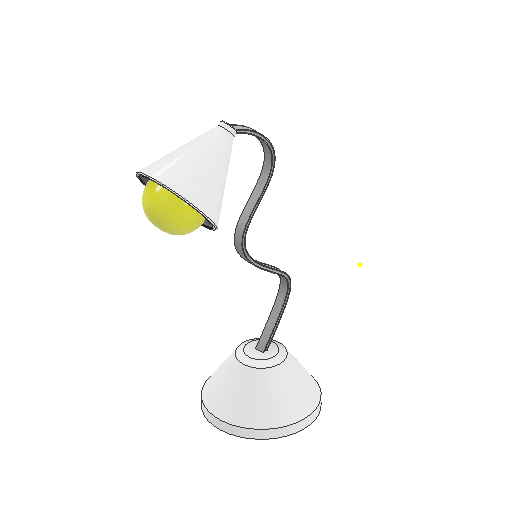
# Autodesk Inventor part: Lamp
Saved by Autodesk Inventor 2026.2 (Build 302298000, 298)
## iProperties
Created: 2026-01-20
Part Number: Lamp
Material: Generic
Document SubType Name: Modeling
Designer: andyeske
Density: 1 g/cm^3
Appearance: Default
Author: andyeske
Autodesk Inventor part; units mm, degrees
ref_plane "YZ Plane" through (0, 0, 0) normal (1, 0, 0) x (0, 1, 0)
ref_plane "XZ Plane" through (0, 0, 0) normal (0, 1, 0) x (-1, 0, 0)
sketch "Sketch1" plane through (0, 0, 0) normal (0, 0, 1) x (1, 0, 0)
  line L0 (0, 0) -> (14.1629, 0)
  line L1 (14.1629, 0) -> (14.1629, 2.8634)
  line L2 (14.1629, 2.8634) -> (5.4597, 15.9183)
  line L3 (5.4597, 15.9183) -> (0, 15.9183)
  line L4 (0, 15.9183) -> (0, 0)
  constraints: 10 end point, 2 perpendicular, 1 horizontal, 1 parallel
revolve "Revolution1" add sketch "Sketch1" angle 360 about axis through (0, 15.9183, 0) along (0, -1, 0)
sketch "Sketch2" plane through (0, 0, 0) normal (1, 0, 0) x (0, 1, 0)
  line L0 (15.9183, 5.4597) -> (15.9183, -5.4597) projected
  spline S0 degree 4 poles (15.9183, 0) (34.1677, -12.4464) (32.4638, -9.3286) (51.0132, 21.4952) (65.6277, -11.3456) (81.7247, 0.6772) (85.1054, 10.9604) (85.0776, 11.7877) knots 0 0 0 0 0 0.334349 0.547583 0.739077 1 1 1 1 1
  line L1 (-0.0819, 10.9124) -> (31.9186, -10.9124) construction
  arc A0 (3.2241, 8.8777) -> (28.8174, -8.5773) centre (387.7406, 545.1818) ccw construction
  line L2 (85.1268, 10.3231) -> (85.0285, 13.2523) construction
  arc A1 (84.8109, 11.3786) -> (84.7841, 12.178) centre (84.6524, 11.7734) ccw construction
  point P0 (0, 0)
  point P1 (37.5795, -3.3142)
  point P2 (52.1302, 7.0993)
  point P3 (67.4583, -2.4293)
  point P4 (81.2439, 4.0296)
  constraints: 5 midpoint, 4 end point, 2 centre point, 2 point on circle, 10 other
sketch "Sketch3" plane through (0, 15.9183, 0) normal (0, 1, 0) x (1, 0, 0)
  line L0 (1.27, -0.635) -> (-1.27, -0.635)
  line L1 (-1.27, -0.635) -> (-1.27, 0.635)
  line L2 (-1.27, 0.635) -> (1.27, 0.635)
  line L3 (1.27, 0.635) -> (1.27, -0.635)
  line L4 (1.27, -0.635) -> (-1.27, 0.635) construction
  line L5 (-1.27, -0.635) -> (1.27, 0.635) construction
  circle A0 centre (-1.27, 0) radius 0.381
  circle A1 centre (1.27, 0) radius 0.381
  point P0 (0, 0)
  point P1 (1.27, -0.381)
  point P2 (1.27, 0.381)
  point P3 (-1.27, 0.381)
  point P4 (-1.27, -0.381)
  dimension "d1" = 2.54
  dimension "d2" = 1.27
  dimension "d3" = 0.762
  dimension "d4" = 0.762
  constraints: 12 end point, 4 midpoint, 2 centre point, 2 parallel, 1 horizontal, 1 perpendicular
  measures "d1" distance of L0.start L0.end
  measures "d2" distance of L0.end L1.end
  measures "d3" diameter of A1
  measures "d4" diameter of A0
sweep "Sweep1" add profiles "Sketch3" path "Sketch2" path curves S0 contours L0 L1 A0 L2 L3 A1
sketch "Sketch4" plane through (-1.27, 85.5899, 12.1629) normal (0, -0.5908599, 0.8067742) x (1, 0, 0)
  line L0 (2.54, 0) -> (0, 0) projected
  line L1 (1.27, 0) -> (1.27, -1.27)
  line L2 (0, -1.27) -> (2.54, -1.27) projected
  line L3 (1.27, -0.635) -> (2.54, -0.635)
  point P0 (1.27, -76.2383)
  constraints: 4 end point, 3 midpoint, 1 horizontal
ref_plane "Work Plane1" through (0, 85.0776, 11.7877) normal (0, -0.8067742, -0.5908599) x (1, 0, 0)
sketch "Sketch5" plane through (0, 85.0776, 11.7877) normal (0, -0.8067742, -0.5908599) x (1, 0, 0)
  line L0 (1.27, 0) -> (-1.27, 0) construction
  line L1 (-1.27, 0) -> (-2.3484, 0)
  line L2 (-2.3484, 0) -> (-11.8168, 20.7123)
  line L3 (-11.8168, 20.7123) -> (0, 20.7123) construction
  line L4 (0, 20.7123) -> (0, 0) construction
  line L5 (-1.27, 0) -> (1.27, 0) projected
  line L6 (0, 0) -> (0, -1.4615)
  line L7 (0, -1.4615) -> (-2.3484, -1.4615)
  line L8 (-2.3484, -1.4615) -> (-2.3484, 0)
  line L9 (-11.8168, 20.7123) -> (-10.5339, 20.7123)
  line L10 (-10.5339, 20.7123) -> (-1.27, 0.7261) construction
  line L11 (-1.27, 0.7261) -> (0, 0.7261) construction
  line L12 (0, -0.4229) -> (0, 0.7261)
  arc A0 (0, 28.1087) -> (-5.2837, 14.8723) centre (-0.7674, 20.7423) ccw
  line L13 (-5.2837, 14.8723) -> (-5.2837, 10.7192)
  line L14 (-5.2837, 10.7192) -> (0, 10.7192) construction
  line L15 (0, 0.7261) -> (0, 28.1087)
  line L16 (-10.5339, 20.7123) -> (-5.9019, 10.7192)
  line L17 (-5.9019, 10.7192) -> (-5.2837, 10.7192)
  point P0 (0, 40.759)
  constraints: 32 end point, 6 point on line, 4 perpendicular, 3 collinear, 2 midpoint, 2 point on circle, 2 vertical, 1 centre point, 1 horizontal, 1 parallel
revolve "Revolution2" add sketch "Sketch5" angle 360 about axis through (0, 72.8396, 28.4979) along (0, 0.5908599, -0.8067742)
fillet "Fillet1" radius 0.254 4 edges at (11.8168, 72.8396, 28.4979) (10.5339, 72.8396, 28.4979) (-1.9566, 84.8934, 9.8412) (1.2987, 87.5197, 11.7647)
chamfer "Chamfer1" distance 1.27 angle 45 1 edges at (-5.4597, 15.9183, 0)
body "Solid1"
